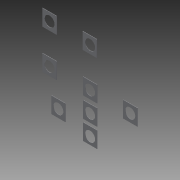
# Autodesk Inventor part: fire_locs
Saved by Autodesk Inventor 2013 (Build 170138000, 138)
## iProperties
Created: 2011-07-25
Part Number: fire_locs
Document SubType Name: Modeling
Designer: rrw
Density: 1 g/cm^3
Material: Generic
Author: rrw
Autodesk Inventor part; units mm, degrees
ref_plane "YZ Plane" through (0, 0, 0) normal (1, 0, 0) x (0, 1, 0)
ref_plane "XZ Plane" through (0, 0, 0) normal (0, 1, 0) x (-1, 0, 0)
ref_plane "XY Plane" through (0, 0, 0) normal (0, 0, 1) x (1, 0, 0)
sketch "Sketch1" plane through (0, 0, 0) normal (0, 0, 1) x (1, 0, 0)
  line L0 (-1412.4225, 1400.3978) -> (-992.4225, 1400.3978)
  line L1 (-992.4225, 1400.3978) -> (-992.4225, 920.3978)
  line L2 (-992.4225, 920.3978) -> (-1412.4225, 920.3978)
  line L3 (-1412.4225, 920.3978) -> (-1412.4225, 1400.3978)
  line L4 (197.4225, 1400.3978) -> (-222.5775, 1400.3978)
  line L5 (-222.5775, 1400.3978) -> (-222.5775, 920.3978)
  line L6 (-222.5775, 920.3978) -> (197.4225, 920.3978)
  line L7 (197.4225, 920.3978) -> (197.4225, 1400.3978)
  line L8 (210, 240) -> (-210, 240)
  line L9 (-210, 240) -> (-210, -240)
  line L10 (-210, -240) -> (210, -240)
  line L11 (210, -240) -> (210, 240)
  line L12 (-1412.4225, 240) -> (-992.4225, 240)
  line L13 (-992.4225, 240) -> (-992.4225, -240)
  line L14 (-992.4225, -240) -> (-1412.4225, -240)
  line L15 (-1412.4225, -240) -> (-1412.4225, 240)
  line L16 (1400.1297, -240) -> (980.1297, -240)
  line L17 (980.1297, -240) -> (980.1297, 240)
  line L18 (980.1297, 240) -> (1400.1297, 240)
  line L19 (1400.1297, 240) -> (1400.1297, -240)
  line L20 (-210, -929.9053) -> (210, -929.9053)
  line L21 (210, -929.9053) -> (210, -1409.9053)
  line L22 (210, -1409.9053) -> (-210, -1409.9053)
  line L23 (-210, -1409.9053) -> (-210, -929.9053)
  line L24 (0, -839.9053) -> (210, -839.9053)
  line L25 (210, -839.9053) -> (-210, -839.9053)
  line L26 (-210, -839.9053) -> (-210, -359.9053)
  line L27 (-210, -359.9053) -> (210, -359.9053)
  line L28 (210, -359.9053) -> (210, -839.9053)
  line L29 (-730.741, -1189.9053) -> (-1150.741, -1189.9053)
  line L30 (-1150.741, -1189.9053) -> (-1150.741, -709.9053)
  line L31 (-1150.741, -709.9053) -> (-730.741, -709.9053)
  line L32 (-730.741, -709.9053) -> (-730.741, -1189.9053)
  circle A0 centre (0, 0) radius 150
  circle A1 centre (0, -599.9053) radius 150
  circle A2 centre (0, -1189.9053) radius 150
  circle A3 centre (-940.741, -949.9053) radius 150
  circle A4 centre (-1202.4225, 0) radius 150
  circle A5 centre (-1202.4225, 1160.3978) radius 150
  circle A6 centre (0, 1160.3978) radius 150
  circle A7 centre (1190.1297, 0) radius 150
  line L33 (-69.7232, -78.3673) -> (0, 98.9981)
  line L34 (0, 98.9981) -> (68.8435, -78.3673)
  line L35 (68.8435, -78.3673) -> (34.4218, 10.3154)
  line L36 (-34.8616, 10.3154) -> (34.4218, 10.3154)
  line L37 (-34.8616, -709.9053) -> (-34.8616, -519.0093)
  line L38 (-34.8616, -519.0093) -> (68.8435, -519.0093)
  line L39 (68.8435, -519.0093) -> (-34.8616, -519.0093)
  line L40 (-34.8616, -614.4573) -> (68.8435, -614.4573)
  line L41 (51.6326, -1099.9053) -> (-69.7232, -1099.9053)
  line L42 (-69.7232, -1099.9053) -> (-69.7232, -1264.2349)
  line L43 (-69.7232, -1264.2349) -> (51.6326, -1264.2349)
  line L44 (51.6326, -1264.2349) -> (51.6326, -1189.9053)
  line L45 (51.6326, -1189.9053) -> (16.991, -1189.9053)
  line L46 (-995.8758, -876.8753) -> (-995.8758, -1039.9053)
  line L47 (-995.8758, -1039.9053) -> (-995.8758, -958.3903)
  line L48 (-875.9765, -876.8753) -> (-875.9765, -1039.9053)
  line L49 (-875.9765, -1039.9053) -> (-875.9765, -968.3774)
  line L50 (-995.8758, -958.3903) -> (-875.9765, -958.3903)
  line L51 (-1245.3239, -90.2242) -> (-1245.3239, 98.9981)
  arc A8 (-1245.3239, -90.2242) -> (-1245.3239, 98.9981) centre (-1225.2999, 4.3869) ccw
  line L52 (1135.9503, 98.9981) -> (1135.9503, -107.8143)
  line L53 (1135.9503, -107.8143) -> (1250.0071, -107.8143)
  line L54 (1250.0071, -107.8143) -> (1135.9503, -107.8143)
  line L55 (1135.9503, -4.4081) -> (1227.555, -4.4081)
  line L56 (1227.555, -4.4081) -> (1135.9503, -4.4081)
  line L57 (1135.9503, 98.9981) -> (1235.6377, 98.9981)
  arc A9 (51.6326, 1265.6539) -> (51.6326, 1054.1252) centre (19.9492, 1159.8895) ccw
  line L58 (-1262.9916, 1259.8929) -> (-1262.9916, 1063.3954)
  arc A10 (-1262.9916, 1161.6442) -> (-1262.9916, 1259.8929) centre (-1246.1479, 1210.7685) ccw
  arc A11 (-1262.9916, 1063.3954) -> (-1262.9916, 1161.6442) centre (-1231.5443, 1112.5198) ccw
  constraints: 118 end point, 25 parallel, 17 perpendicular, 12 centre point, 8 horizontal, 8 point on circle, 7 midpoint, 2 collinear, 1 coincident, 1 point on line
extrude "Extrusion1" add sketch "Sketch1" along normal blind 10 contours L0 L1 L2 L3 | L7 L6 L5 L4 | L11 L10 L9 L8 | L12 L13 L14 L15 | L16 L17 L18 L19 | L20 L21 L22 L23 | L25 L26 L27 L28 L24 | L29 L30 L31 L32
body "Solid1"
